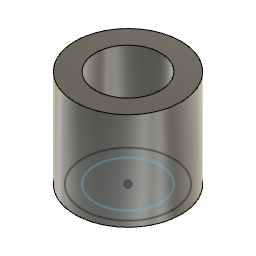
PCB Tube-6.0mm v1 (Autodesk Fusion 360 design; units mm, degrees)
Autodesk Fusion 360 part; units mm, degrees
sketch "Sketch1" plane through (0, 0, 0) normal (0, 0, 1) x (1, 0, 0)
  circle A0 centre (0, 0) radius 2
  circle A1 centre (0, 0) radius 2.75
  dimension "d5" = 4
  dimension "d8" = 5.5
  constraint coincident A0.centre A1.centre
  measures "d5" diameter of A0
  measures "d8" diameter of A1
extrude "Extrude2" add sketch "Sketch1" along normal blind 6.6
move_face "OffsetFaces1" offset 0.5 1 faces at (2.7466, -0.1371, 4.4)
extrude "Extrude3" cut 1 faces at (2.8212, 0.1615, 6.6) along direction (0, 0, -1) blind 1.6
extrude "Extrude4" add 1 faces at (2.8212, 0.1615, 5) along direction (0, 0, 1) blind 1
